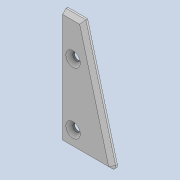
# Autodesk Inventor part: spazzola - appoggio
Saved by Autodesk Inventor 2022 (Build 260153000, 153)
## iProperties
Created: 2025-08-21
Part Number: spazzola - appoggio
Material: Generic
Document SubType Name: Modeling
Designer: 1234
Density: 1 g/cm^3
Appearance: Default
Author: 1234
Autodesk Inventor part; units mm, degrees
ref_plane "YZ Plane" through (0, 0, 0) normal (1, 0, 0) x (0, 1, 0)
ref_plane "XZ Plane" through (0, 0, 0) normal (0, 1, 0) x (-1, 0, 0)
ref_plane "XY Plane" through (0, 0, 0) normal (0, 0, 1) x (1, 0, 0)
sketch "Sketch1" plane through (0, 0, 0) normal (0, 0, 1) x (1, 0, 0)
  line L0 (0, 0) -> (0, 60)
  line L1 (0, 60) -> (9, 60) construction
  line L2 (9, 60) -> (25, 0) construction
  line L3 (25, 0) -> (0, 0) construction
  line L4 (28.2341, -0.4847) -> (11.3048, 63)
  line L5 (11.3048, 63) -> (-3, 63)
  line L6 (-3, 63) -> (-3, -3)
  line L7 (-3, -3) -> (26.3016, -3)
  line L8 (0, 60) -> (0, 63)
  line L9 (0, 0) -> (0, -3)
  arc A0 (26.3016, -3) -> (28.2341, -0.4847) centre (26.3016, -1) ccw
  point P0 (28.9048, -3)
  dimension "d0" = 9
  dimension "d1" = 25
  dimension "d2" = 60
  dimension "d5" = 3
  dimension "d19" = 2
  constraints: 20 end point, 4 point on line, 3 perpendicular, 2 parallel, 2 point on circle, 2 tangent, 2 vertical, 1 centre point, 3 other
  measures "d0" distance of L0.end L1.end
  measures "d1" distance of L2.end L0.start
  measures "d2" distance of L0.start L0.end
  measures "d5" distance between parallel lines of L2 L4
  measures "d19" radius of A0
extrude "Extrusion1" add sketch "Sketch1" along normal blind 3 contours L0 L8 L5 L4 A0 L7 L9
chamfer "Chamfer1" distance 2 angle 45 3 edges at (19.7695, 31.2577, 3) (5.6524, 63, 3) (13.1508, -3, 3)
sketch "Sketch2" plane through (0, 0, 3) normal (0, 0, 1) x (1, 0, 0)
  line L0 (6, -14.251) -> (6, 80.2953) construction
  line L1 (0, 61) -> (0, -1) projected
  circle A0 centre (6, 7) radius 2.1
  circle A1 centre (6, 42) radius 2.1
  line L2 (0, -3) -> (26.3016, -3) projected
  point P0 (0, 0)
  point P1 (28.8571, -3)
  dimension "d9" = 6
  dimension "d10" = 4.2
  dimension "d11" = 4.2
  dimension "d12" = 10
  dimension "d13" = 45
  constraints: 2 centre point, 2 end point, 2 point on line, 1 vertical
  measures "d9" distance between parallel lines of L1 L0
  measures "d10" diameter of A1
  measures "d11" diameter of A0
  measures "d12" distance from line of L2 A0.centre
  measures "d13" distance from line of L2 A1.centre
extrude "Extrusion2" cut sketch "Sketch2" against normal up to surface (3 mm away)
chamfer "Chamfer2" distance 2 angle 45 2 edges at (3.9, 42, 3) (3.9, 7, 3)
equation "\"d11\" = d10"
body "Solid1"
